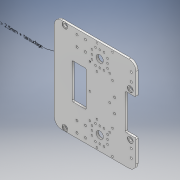
# Autodesk Inventor part: new_torso_middleplate_nuc
Saved by Autodesk Inventor 2018 (Build 220112000, 112)
## iProperties
Created: 2017-02-16
Part Number: new_torso_middleplate_nuc
Material: Aluminum 2014-T4
Document SubType Name: Modeling
Designer: steve
Mass: 110.588 g
Surface Area: 299.466 cm^2
Volume: 39.4957 cm^3
Density: 2.8 g/cm^3
Appearance: Satin
Vendor: Rhoban
Author: steve
Autodesk Inventor part; units mm, degrees
ref_plane "YZ Plane" through (0, 0, 0) normal (1, 0, 0) x (0, 1, 0)
ref_plane "XZ Plane" through (0, 0, 0) normal (0, 1, 0) x (-1, 0, 0)
ref_plane "XY Plane" through (0, 0, 0) normal (0, 0, 1) x (1, 0, 0)
derived "new_torso_topplate.ipt"
sketch "Sketch1" plane through (0, 0, 0) normal (0, 1, 0) x (-1, 0, 0)
  line L0 (-41, 66.5) -> (41, 66.5) construction
  line L1 (41, 66.5) -> (41, -66.5) construction
  line L2 (41, -66.5) -> (-41, -66.5) construction
  line L3 (-41, -66.5) -> (-41, 66.5) construction
  line L4 (-41, 66.5) -> (41, -66.5) construction
  line L5 (41, 66.5) -> (-41, -66.5) construction
  line L6 (106.5296, 0) -> (-65.5883, 0) construction
  line L7 (66.5, -42.5) -> (61.25, -42.5) construction
  line L8 (41, -42.5) -> (41, 42.5) construction
  line L9 (41, 42.5) -> (66.5, 42.5) construction
  line L10 (66.5, 42.5) -> (66.5, -42.5) construction
  line L11 (66.5, -42.5) -> (41, 42.5) construction
  line L12 (41, -42.5) -> (66.5, 42.5) construction
  line L13 (74, 66.5) -> (74, -66.5) construction
  line L14 (-41, 66.5) -> (74, 66.5)
  line L15 (74, 66.5) -> (74, -66.5)
  line L16 (74, -66.5) -> (-41, -66.5)
  line L17 (-41, -66.5) -> (-41, 66.5)
  circle A0 centre (65.4393, 41.4393) radius 1.5 construction
  line L18 (66.5, 42.5) -> (60.0868, 36.0868) construction
  line L19 (66.5, 42.5) -> (75.5696, 42.5) construction
  line L20 (66.5, -42.5) -> (64.7221, -40.7221) construction
  line L21 (66.5, -42.5) -> (69.0143, -42.5) construction
  line L22 (41, -42.5) -> (42.6048, -40.8952) construction
  line L23 (41, -42.5) -> (43.2695, -42.5) construction
  line L24 (41, 42.5) -> (46.0799, 37.4201) construction
  line L25 (41, 42.5) -> (48.184, 42.5) construction
  circle A1 centre (42.0607, 41.4393) radius 1.5 construction
  circle A2 centre (65.4393, -41.4393) radius 1.5 construction
  circle A3 centre (42.0607, -41.4393) radius 1.5 construction
  line L26 (43.1213, 42.5) -> (46.25, 42.5)
  line L27 (66.5, 40.3787) -> (66.5, -40.3787)
  line L28 (64.3787, -42.5) -> (61.25, -42.5)
  line L29 (41, -40.3787) -> (41, 40.3787)
  arc A4 (66.5, 40.3787) -> (64.3787, 42.5) centre (65.4393, 41.4393) ccw
  arc A5 (64.3787, -42.5) -> (66.5, -40.3787) centre (65.4393, -41.4393) ccw
  arc A6 (41, -40.3787) -> (43.1213, -42.5) centre (42.0607, -41.4393) ccw
  arc A7 (43.1213, 42.5) -> (41, 40.3787) centre (42.0607, 41.4393) ccw
  line L30 (81.9414, -45.5) -> (23.4915, -45.5) construction
  line L31 (53.75, 61.7827) -> (53.75, -107.6212) construction
  line L32 (46.25, -34.6173) -> (61.25, -34.6173) construction
  line L33 (61.25, -34.6173) -> (61.25, -50.3827) construction
  line L34 (61.25, -50.3827) -> (46.25, -50.3827) construction
  line L35 (46.25, -50.3827) -> (46.25, -34.6173) construction
  line L36 (46.25, -34.6173) -> (61.25, -50.3827) construction
  line L37 (61.25, -34.6173) -> (46.25, -50.3827) construction
  arc A8 (46.25, -42.5) -> (61.25, -42.5) centre (53.75, -34.625) ccw
  line L38 (61.25, -42.5) -> (41, -42.5) construction
  line L39 (61.25, -42.5) -> (46.25, -42.5) construction
  line L40 (46.25, -42.5) -> (43.1213, -42.5)
  arc A9 (61.25, 42.5) -> (46.25, 42.5) centre (53.75, 34.625) ccw
  line L41 (61.25, 42.5) -> (64.3787, 42.5)
  line L42 (46.25, 42.5) -> (61.25, 42.5) construction
  line L43 (64.3787, 42.5) -> (66.5, 42.5)
  line L44 (66.5, 42.5) -> (66.5, 40.3787)
  line L45 (64.3787, -42.5) -> (66.5, -42.5)
  line L46 (66.5, -42.5) -> (66.5, -40.3787)
  point P0 (0, 0)
  point P1 (53.75, 0)
  point P2 (53.75, 0)
  point P3 (53.75, -42.5)
sketch "Sketch2" plane through (0, 3, 0) normal (0, 1, 0) x (1, 0, 0)
  arc A0 (-74, -56.5) -> (-64, -66.5) centre (-64, -56.5) ccw construction
  line L0 (-64, -66.5) -> (31, -66.5) construction
  arc A1 (31, -66.5) -> (41, -56.5) centre (31, -56.5) ccw construction
  line L1 (41, -56.5) -> (41, 56.5) construction
  arc A2 (41, 56.5) -> (31, 66.5) centre (31, 56.5) ccw construction
  line L2 (31, 66.5) -> (-64, 66.5) construction
  arc A3 (-64, 66.5) -> (-74, 56.5) centre (-64, 56.5) ccw construction
  line L3 (-74, 56.5) -> (-74, -56.5) construction
  line L4 (-66.5, -42.5) -> (-66.5, 42.5) construction
  line L5 (-66.5, 42.5) -> (-61.25, 42.5) construction
  arc A4 (-41, 40.3787) -> (-43.1213, 42.5) centre (-42.0607, 41.4393) ccw construction
  line L6 (-41, 40.3787) -> (-41, -40.3787) construction
  arc A5 (-43.1213, -42.5) -> (-41, -40.3787) centre (-42.0607, -41.4393) ccw construction
  line L7 (-43.1213, -42.5) -> (-46.25, -42.5) construction
  line L8 (31.25, -56.5) -> (37.5, -56.5) construction
  line L9 (37.5, -56.5) -> (37.5, -36.5) construction
  line L10 (37.5, -36.5) -> (31.25, -36.5) construction
  line L11 (31.25, -36.5) -> (31.25, -56.5) construction
  line L12 (37.5, 78) -> (37.5, -82) construction
  line L13 (41, -56.5) -> (-13.5, -56.5) construction
  line L14 (41, -56.5) -> (41, 56.5) construction
  line L15 (41, 56.5) -> (10.5, 56.5) construction
  line L16 (37.5, 56.5) -> (31.25, 56.5) construction
  line L17 (31.25, 56.5) -> (31.25, 36.5) construction
  line L18 (31.25, 36.5) -> (37.5, 36.5) construction
  line L19 (37.5, 36.5) -> (37.5, 56.5) construction
  line L20 (34.375, -36.5) -> (34.375, -56.5) construction
  line L21 (34.375, 36.5) -> (34.375, 56.5) construction
  line L22 (31.25, 46.5) -> (48, 46.5) construction
  line L23 (31.25, -46.5) -> (52, -46.5) construction
  line L24 (-75, -63) -> (42, -63) construction
  line L25 (-71, 63) -> (42, 63) construction
  line L26 (-46, -105.44) -> (-46, 104.2053) construction
  line L27 (-41, 40.3787) -> (-41, -40.3787) construction
  line L28 (-46, -63) -> (-26, -63) construction
  line L29 (-26, -63) -> (-26, -56.75) construction
  line L30 (-26, -56.75) -> (-46, -56.75) construction
  line L31 (-46, -56.75) -> (-46, -63) construction
  line L32 (-46, -59.875) -> (-26, -59.875) construction
  line L33 (-36, -56.75) -> (-36, -63) construction
  line L34 (-46, 63) -> (-46, 56.75) construction
  line L35 (-36, 63) -> (-36, 56.75) construction
  line L36 (-26, 63) -> (-46, 63) construction
  line L37 (-46, 59.875) -> (-26, 59.875) construction
  line L38 (-46, 56.75) -> (-26, 56.75) construction
  line L39 (-26, 56.75) -> (-26, 63) construction
  arc A6 (-61.25, -42.5) -> (-46.25, -42.5) centre (-53.75, -34.625) ccw
  line L40 (-61.25, -42.5) -> (-66.5, -42.5)
  arc A7 (-46.25, 42.5) -> (-61.25, 42.5) centre (-53.75, 34.625) ccw
  line L41 (-46.25, 42.5) -> (-43.1213, 42.5)
  point P0 (0, 0)
  point P1 (34.375, -52.5)
  point P2 (34.375, -40.5)
  point P3 (34.375, 40.5)
  point P4 (34.375, 52.5)
  point P5 (-30, 59.875)
  point P6 (-42, 59.875)
  point P7 (-30, -59.875)
  point P8 (-42, -59.875)
extrude "Extrusion1" add sketch "Sketch1" along normal blind 3 contours L14 L15 L16 L17 | L26 A9 L41 L43 L44 L27 L46 L45 L28 A8 L40 A6 L29 A7 | A4 L43 | A4 L44 | A5 L46 | L45 A5
hole "Hole1" at (34.375, 3, 52.5) at (34.375, 3, 40.5) at (34.375, 3, -40.5) at (34.375, 3, -52.5) at (-30, 3, -59.875) at (-42, 3, -59.875) at (-30, 3, 59.875) at (-42, 3, 59.875) direction (0, -1, 0) diameter 3 end through all countersink diameter 4 countersink angle 90
fillet "Fillet1" radius 10 4 edges at (41, 1.5, -66.5) (-74, 1.5, -66.5) (-74, 1.5, 66.5) (41, 1.5, 66.5)
sketch "Sketch3" plane through (-64, 3, -66.5) normal (0, 1, 0) x (1, 0, 0)
  line L0 (54.127, -146) -> (54.127, 14) construction
  line L1 (-10, -10) -> (-10, -123) construction
  line L2 (-10, -66.5) -> (90, -66.5) construction
  line L3 (-17, -20.125) -> (94, -20.125) construction
  circle A0 centre (54.127, -20.125) radius 5
  circle A1 centre (54.127, -112.875) radius 5
  line L4 (105, -123) -> (105, -10) projected
  point P0 (64, -66.5)
  dimension "d12" = 46.375
  dimension "d13" = 10
  dimension "d90" = 50.873
  constraints: 6 end point, 2 centre point, 2 horizontal, 2 point on line, 1 midpoint, 1 symmetric about line, 1 vertical, 1 other
  measures "d12" distance between parallel lines of L3 L2
  measures "d13" diameter of A0
  measures "d90" distance between parallel lines of L4 L0
extrude "Extrusion2" cut sketch "Sketch3" against normal blind 3
sketch "Sketch4" plane through (-64, 3, -66.5) normal (0, 1, 0) x (1, 0, 0)
  line L0 (-10, -10) -> (-10, -123) construction
  line L1 (-10, -66.5) -> (105, -66.5) construction
  line L2 (105, -123) -> (105, -10) construction
  circle A0 centre (54.127, -20.125) radius 5 construction
  circle A1 centre (54.127, -20.125) radius 12.53 construction
  line L3 (65.127, -14.125) -> (43.127, -14.125) construction
  line L4 (43.127, -14.125) -> (43.127, -26.125) construction
  line L5 (43.127, -26.125) -> (65.127, -26.125) construction
  line L6 (65.127, -26.125) -> (65.127, -14.125) construction
  line L7 (65.127, -14.125) -> (43.127, -26.125) construction
  line L8 (43.127, -14.125) -> (65.127, -26.125) construction
  line L9 (60.127, -9.125) -> (48.127, -9.125) construction
  line L10 (48.127, -9.125) -> (48.127, -31.125) construction
  line L11 (48.127, -31.125) -> (60.127, -31.125) construction
  line L12 (60.127, -31.125) -> (60.127, -9.125) construction
  line L13 (60.127, -9.125) -> (48.127, -31.125) construction
  line L14 (48.127, -9.125) -> (60.127, -31.125) construction
  circle A2 centre (54.127, -112.875) radius 5 construction
  circle A3 centre (54.127, -112.875) radius 12.53 construction
  line L15 (65.127, -118.875) -> (43.127, -118.875) construction
  line L16 (43.127, -118.875) -> (43.127, -106.875) construction
  line L17 (43.127, -106.875) -> (65.127, -106.875) construction
  line L18 (65.127, -106.875) -> (65.127, -118.875) construction
  line L19 (65.127, -118.875) -> (43.127, -106.875) construction
  line L20 (43.127, -118.875) -> (65.127, -106.875) construction
  line L21 (60.127, -123.875) -> (48.127, -123.875) construction
  line L22 (48.127, -123.875) -> (48.127, -101.875) construction
  line L23 (48.127, -101.875) -> (60.127, -101.875) construction
  line L24 (60.127, -101.875) -> (60.127, -123.875) construction
  line L25 (60.127, -123.875) -> (48.127, -101.875) construction
  line L26 (48.127, -123.875) -> (60.127, -101.875) construction
  circle A4 centre (54.127, -20.125) radius 11 construction
  line L27 (54.127, -1.5995) -> (54.127, -39.9214) construction
  line L28 (69.9841, -20.125) -> (35.4491, -20.125) construction
  line L29 (72.127, -2.825) -> (50.127, -2.825) construction
  line L30 (50.127, -2.825) -> (50.127, -37.425) construction
  line L31 (50.127, -37.425) -> (72.127, -37.425) construction
  line L32 (72.127, -37.425) -> (72.127, -2.825) construction
  line L33 (72.127, -20.125) -> (50.127, -20.125) construction
  point P0 (64, -66.5)
  point P1 (54.127, -20.125)
  point P2 (54.127, -9.125)
  point P3 (65.127, -20.125)
  point P4 (54.127, -31.125)
  point P5 (43.127, -20.125)
  point P6 (54.127, -123.875)
  point P7 (65.127, -112.875)
  point P8 (54.127, -101.875)
  point P9 (43.127, -112.875)
  point P10 (72.127, -130.175)
  point P11 (72.127, -95.575)
  point P12 (50.127, -95.575)
  point P13 (50.127, -130.175)
  dimension "d16" = 25.06
  dimension "d17" = 12
  dimension "d18" = 12
  dimension "d31" = 22
  dimension "d32" = 34.6
  dimension "d33" = 22
  dimension "d34" = 4
  constraints: 64 end point, 26 symmetric about line, 21 coincident, 14 midpoint, 8 point on circle, 6 parallel, 6 point on line, 4 centre point, 4 horizontal, 3 perpendicular, 1 collinear, 1 concentric, 1 vertical, 2 other
  measures "d16" diameter of A1
  measures "d17" distance of L3.end L4.end
  measures "d18" distance of L10.end L11.end
  measures "d31" diameter of A4
  measures "d32" distance of L29.end L30.end
  measures "d33" distance of L29.start L29.end
  measures "d34" distance between parallel lines of L27 L30
hole "Hole2" at (-20.873, 3, -40.375) at (-20.873, 3, -52.375) at (-15.873, 3, -57.375) at (-3.873, 3, -57.375) at (1.127, 3, -52.375) at (1.127, 3, -40.375) at (-3.873, 3, -35.375) at (-15.873, 3, -35.375) at (-15.873, 3, 35.375) at (-3.873, 3, 35.375) at (1.127, 3, 40.375) at (1.127, 3, 52.375) at (-3.873, 3, 57.375) at (-15.873, 3, 57.375) at (-20.873, 3, 52.375) at (-20.873, 3, 40.375) at (1.127, 3, -46.375) at (-9.873, 3, -57.375) at (-20.873, 3, -46.375) at (-9.873, 3, -35.375) at (1.127, 3, 46.375) at (-9.873, 3, 35.375) at (-20.873, 3, 46.375) at (-9.873, 3, 57.375) at (8.127, 3, -29.075) at (8.127, 3, -63.675) at (-13.873, 3, -29.075) at (-13.873, 3, -63.675) at (8.127, 3, 29.075) at (8.127, 3, 63.675) at (-13.873, 3, 63.675) at (-13.873, 3, 29.075) direction (0, -1, 0) diameter 2.5 end through all
sketch "Sketch5" plane through (-64, 0, 66.5) normal (0, -1, 0) x (1, 0, 0)
  line L0 (68.127, -66.5) -> (40.127, -66.5) construction
  line L1 (40.127, -66.5) -> (40.127, -102.5) construction
  line L2 (40.127, -102.5) -> (68.127, -102.5) construction
  line L3 (68.127, -102.5) -> (68.127, -66.5) construction
  line L4 (72.127, -9.5) -> (36.127, -9.5) construction
  line L5 (36.127, -9.5) -> (36.127, -106.5) construction
  line L6 (36.127, -106.5) -> (72.127, -106.5) construction
  line L7 (72.127, -106.5) -> (72.127, -9.5) construction
  line L8 (54.127, -66.5) -> (54.127, -102.5) construction
  line L9 (54.127, -9.5) -> (54.127, -106.5) construction
  circle A0 centre (54.127, -20.125) radius 5 projected
  line L10 (105, -10) -> (105, -123) construction
  line L11 (105, -66.5) -> (-10, -66.5) construction
  line L12 (-10, -123) -> (-10, -10) construction
  point P0 (64, -66.5)
  point P1 (68.127, -30.5)
  point P2 (40.127, -30.5)
  dimension "d26" = 28
  dimension "d27" = 36
  dimension "d28" = 97
  dimension "d29" = 36
  dimension "d30" = 4
  constraints: 22 end point, 6 midpoint, 4 coincident, 4 parallel, 2 horizontal, 2 perpendicular, 2 point on line, 2 symmetric about line, 1 collinear
  measures "d26" distance of L1.end L2.end
  measures "d27" distance of L0.end L1.end
  measures "d28" distance of L6.end L4.start
  measures "d29" distance of L5.end L6.end
  measures "d30" distance between parallel lines of L6 L2
hole "Hole3" at (4.127, 0, -36) at (-23.873, 0, -36) at (-23.873, 0, 0) at (4.127, 0, 0) at (-23.873, 0, 36) at (4.127, 0, 36) direction (0, 1, 0) diameter 2.5 end through all
sketch "Sketch6" plane through (-64, 0, 66.5) normal (0, -1, 0) x (1, 0, 0)
  line L0 (105, -10) -> (105, -123) construction
  line L1 (105, -66.5) -> (-44.6068, -66.5) construction
  line L2 (90, -41.5) -> (105, -41.5)
  line L3 (105, -41.5) -> (105, -91.5)
  line L4 (105, -91.5) -> (90, -91.5)
  line L5 (90, -91.5) -> (90, -41.5)
  line L6 (90, -41.5) -> (105, -91.5) construction
  line L7 (105, -41.5) -> (90, -91.5) construction
  point P0 (64, -66.5)
  point P1 (97.5, -66.5)
  dimension "d42" = 15
  dimension "d43" = 50
  constraints: 14 end point, 3 midpoint, 2 horizontal, 2 parallel, 2 point on line, 1 perpendicular
  measures "d42" distance between parallel lines of L0 L5
  measures "d43" distance between parallel lines of L4 L2
extrude "Extrusion3" cut sketch "Sketch6" against normal through all
fillet "Fillet2" radius 1.5 4 edges at (41, 1.5, -25) (26, 1.5, -25) (26, 1.5, 25) (41, 1.5, 25)
sketch "Sketch7" plane through (-64, 0, 66.5) normal (0, -1, 0) x (1, 0, 0)
  line L0 (-10, -123) -> (-10, -10) construction
  line L1 (-10, -66.5) -> (114.3299, -66.5) construction
  line L2 (15, -91.5) -> (35, -91.5)
  line L3 (35, -91.5) -> (35, -41.5)
  line L4 (35, -41.5) -> (15, -41.5)
  line L5 (15, -41.5) -> (15, -91.5)
  line L6 (15, -91.5) -> (35, -41.5) construction
  line L7 (35, -91.5) -> (15, -41.5) construction
  line L8 (91.5, -41.5) -> (103.5, -41.5) projected
  point P0 (64, -66.5)
  point P1 (25, -66.5)
  dimension "d47" = 20
  dimension "d48" = 25
  constraints: 14 end point, 3 midpoint, 2 horizontal, 2 parallel, 1 collinear, 1 perpendicular, 1 point on line
  measures "d47" distance of L2.start L2.end
  measures "d48" distance between parallel lines of L5 L0
extrude "Extrusion4" cut sketch "Sketch7" against normal through all
fillet "Fillet3" radius 1.5 4 edges at (-29, 1.5, 25) (-29, 1.5, -25) (-49, 1.5, -25) (-49, 1.5, 25)
sketch "Sketch8" plane through (-64, 0, 66.5) normal (0, -1, 0) x (1, 0, 0)
  circle A0 centre (97, -35.5) radius 5 construction
  line L0 (102, 18.8567) -> (102, -57.8576) construction
  line L1 (105, -10) -> (105, -40) construction
  line L2 (103.5, -41.5) -> (91.5, -41.5) construction
  arc A1 (0, 0) -> (-10, -10) centre (0, -10) ccw construction
  circle A2 centre (5, -4) radius 4 construction
  line L3 (49.3756, 0) -> (1.1432, 0) construction
  line L4 (0, 0) -> (95, 0) construction
  line L5 (-10, -123) -> (-10, -10) construction
  line L6 (-10, -66.5) -> (151.1007, -66.5) construction
  circle A3 centre (97, -97.5) radius 5 construction
  circle A4 centre (5, -129) radius 4 construction
  line L7 (5, 23.5385) -> (5, -34.4005) construction
  line L8 (1, 8.2413) -> (1, -29.9928) construction
  point P0 (64, -66.5)
  dimension "d52" = 10
  dimension "d53" = 3
  dimension "d54" = 6
  dimension "d56" = 8
  dimension "d57" = 0
  dimension "d65" = 15
  constraints: 10 end point, 5 centre point, 4 coincident, 4 symmetric about line, 3 tangent, 3 vertical, 2 horizontal, 2 point on circle, 1 midpoint, 1 point on line, 2 other
  measures "d52" diameter of A0
  measures "d53" distance between parallel lines of L0 L1
  measures "d54" distance from line of L2 A0.centre
  measures "d56" diameter of A2
  measures "d57" distance between parallel lines of L4 L3
  measures "d65" distance between parallel lines of L7 L5
hole "Hole4" at (33, 0, 31) at (-59, 0, 62.5) at (33, 0, -31) at (-59, 0, -62.5) direction (0, 1, 0) diameter 5 end through all
sketch "Sketch9" plane through (-64, 3, -66.5) normal (0, 1, 0) x (1, 0, 0)
  line L0 (-10, -10) -> (-10, -123) construction
  line L1 (-10, -66.5) -> (119.2694, -66.5) construction
  line L2 (75, -155.2566) -> (75, 35.5463) construction
  line L3 (90, -90) -> (90, -43) construction
  point P0 (64, -66.5)
  point P1 (75, -76.5)
  point P2 (75, -56.5)
  dimension "d66" = 15
  dimension "d74" = 10
  constraints: 4 end point, 1 horizontal, 1 midpoint, 1 point on line, 1 symmetric about line, 1 vertical
  measures "d66" distance between parallel lines of L3 L2
  measures "d74" distance from line of L1 point (75, -76.5)
hole "Hole5" at (11, 3, 10) at (11, 3, -10) direction (0, -1, 0) diameter 3 end through all
sketch "Sketch10" plane through (-64, 0, 66.5) normal (0, -1, 0) x (1, 0, 0)
  circle A0 centre (5, -4) radius 2.5 projected
  circle A1 centre (97, -35.5) radius 2.5 projected
  circle A2 centre (5, -129) radius 2.5 projected
  circle A3 centre (97, -97.5) radius 2.5 projected
  circle A4 centre (5, -4) radius 4.05
  circle A5 centre (5, -129) radius 4.05
  circle A6 centre (97, -97.5) radius 4.05
  circle A7 centre (97, -35.5) radius 4.05
  point P0 (64, -66.5)
  dimension "d75" = 8.1
  dimension "d76" = 8.1
  dimension "d77" = 8.1
  dimension "d78" = 8.1
  constraints: 4 centre point, 4 coincident
  measures "d75" diameter of A4
  measures "d76" diameter of A5
  measures "d77" diameter of A6
  measures "d78" diameter of A7
extrude "Extrusion5" cut sketch "Sketch10" against normal blind 0.5
sketch "Sketch11" plane through (-64, 0, 66.5) normal (0, -1, 0) x (1, 0, 0)
  line L0 (-24.7602, -111.375) -> (131.0452, -111.375) construction
  line L1 (-74.4483, -21.625) -> (173.9542, -21.625) construction
  line L2 (-24.7602, -126.375) -> (132.4394, -126.375) construction
  line L3 (131.0452, -6.625) -> (-33.335, -6.625) construction
  line L4 (22, 29.1448) -> (22, -148.124) construction
  line L5 (34, 27.6122) -> (34, -148.124) construction
  circle A0 centre (22, -6.625) radius 1.5 construction
  circle A1 centre (34, -6.625) radius 1.5 construction
  circle A2 centre (22, -126.375) radius 1.5 construction
  circle A3 centre (34, -126.375) radius 1.5 construction
  point P0 (64, -66.5)
  point P1 (22, -21.625)
  point P2 (34, -21.625)
  point P3 (22, -111.375)
  point P4 (34, -111.375)
  dimension "d81" = 15
  dimension "d82" = 15
  constraints: 12 end point, 12 point on line, 4 horizontal, 2 vertical
  measures "d81" distance between parallel lines of L0 L2
  measures "d82" distance between parallel lines of L3 L1
hole "Hole6" at (-42, 0, 44.875) at (-30, 0, 44.875) at (-42, 0, -44.875) at (-30, 0, -44.875) direction (0, 1, 0) diameter 3 end through all
equation "\"d1\" = torso_topplate_d"
equation "\"d14\" = torso_topplate_d"
equation "\"torso_topplate_d\" = 3"
body "Solid1"
